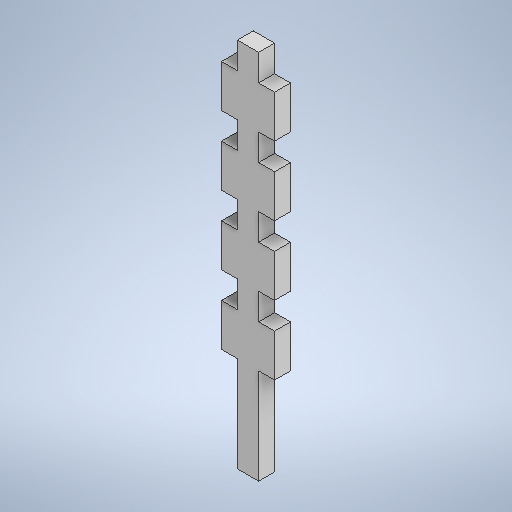
# Autodesk Inventor part: select holder pt 3
Saved by Autodesk Inventor 2025.3 (Build 293356000, 356)
## iProperties
Created: 2026-04-27
Part Number: select holder pt 3
Material: Generic
Document SubType Name: Modeling
Designer: kamal
Density: 1 g/cm^3
Appearance: Default
Author: kamal
Autodesk Inventor part; units mm, degrees
ref_plane "YZ Plane" through (0, 0, 0) normal (1, 0, 0) x (0, 1, 0)
ref_plane "XZ Plane" through (0, 0, 0) normal (0, 1, 0) x (-1, 0, 0)
ref_plane "XY Plane" through (0, 0, 0) normal (0, 0, 1) x (1, 0, 0)
sketch "Sketch1" plane through (0, 0, 0) normal (0, 0, 1) x (1, 0, 0)
  line L0 (0, 0) -> (0, 70) construction
  line L1 (0, 70) -> (-2, 70)
  line L2 (-2, 70) -> (-2, 65)
  line L3 (-2, 65) -> (-5, 65)
  line L4 (-5, 65) -> (-5, 57)
  line L5 (-5, 57) -> (-2, 57)
  line L6 (-2, 57) -> (-2, 52)
  line L7 (-2, 52) -> (-5, 52)
  line L8 (-5, 52) -> (-5, 44)
  line L9 (-5, 44) -> (-2, 44)
  line L10 (-2, 44) -> (-2, 39)
  line L11 (-2, 39) -> (-5, 39)
  line L12 (-5, 39) -> (-5, 31)
  line L13 (-5, 31) -> (-2, 31)
  line L14 (-2, 31) -> (-2, 26)
  line L15 (-2, 26) -> (-5, 26)
  line L16 (-5, 26) -> (-5, 18)
  line L17 (-5, 18) -> (-2, 18)
  line L18 (-2, 18) -> (-2, 0)
  line L19 (-2, 0) -> (0, 0)
  line L20 (0, 70) -> (2, 70)
  line L21 (2, 70) -> (2, 65)
  line L22 (2, 65) -> (5, 65)
  line L23 (5, 65) -> (5, 57)
  line L24 (5, 57) -> (2, 57)
  line L25 (2, 57) -> (2, 52)
  line L26 (5, 52) -> (5, 44)
  line L27 (5, 44) -> (2, 44)
  line L28 (2, 44) -> (2, 39)
  line L29 (2, 39) -> (5, 39)
  line L30 (5, 39) -> (5, 31)
  line L31 (5, 31) -> (2, 31)
  line L32 (2, 31) -> (2, 26)
  line L33 (5, 26) -> (5, 18)
  line L34 (5, 18) -> (2, 18)
  line L35 (2, 18) -> (2, 0)
  line L36 (2, 0) -> (0, 0)
  line L37 (5, 52) -> (2, 52)
  line L38 (5, 26) -> (2, 26)
  dimension "d2" = 70
  dimension "d3" = 2
  dimension "d4" = 5
  dimension "d5" = 3
  dimension "d6" = 8
  dimension "d7" = 3
  dimension "d8" = 5
  dimension "d9" = 8
  dimension "d10" = 5
  dimension "d11" = 8
  dimension "d12" = 3
  dimension "d13" = 5
  dimension "d14" = 3
  dimension "d15" = 8
  dimension "d16" = 4
  constraints: 78 end point, 20 point on line, 18 symmetric about line, 7 perpendicular, 5 horizontal, 2 vertical, 1 parallel
  measures "d2" distance of L0.start L0.end
  measures "d3" distance of L0.end L1.end
  measures "d4" distance of L1.end L2.end
  measures "d5" distance of L2.end L3.end
  measures "d6" distance of L3.end L4.end
  measures "d7" distance of L4.end L5.end
  measures "d8" distance of L5.end L6.end
  measures "d9" distance of L7.end L8.end
  measures "d10" distance of L9.end L10.end
  measures "d11" distance of L11.end L12.end
  measures "d12" distance of L12.end L13.end
  measures "d13" distance of L13.end L14.end
  measures "d14" distance of L14.end L15.end
  measures "d15" distance of L15.end L16.end
  measures "d16" diameter of L10 L0
extrude "Extrusion1" add sketch "Sketch1" along normal blind 3
body "Solid1"
